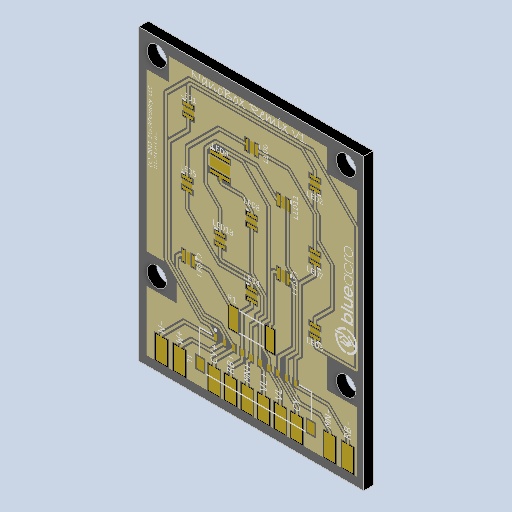
# Autodesk Inventor part: nanobox_v31_upgrade_BOARD
Saved by Autodesk Inventor 2023.2 (Build 272271030, 271C)
## iProperties
Created: 2023-03-08
Part Number: nanobox_v31_upgrade_BOARD
Material: Generic
Document SubType Name: Modeling
Designer: atrus
Density: 1 g/cm^3
Appearance: BoardColor
Author: atrus
Autodesk Inventor part; units mm, degrees
ref_plane "YZ Plane" through (0, 0, 0) normal (1, 0, 0) x (0, 1, 0)
ref_plane "XZ Plane" through (0, 0, 0) normal (0, 1, 0) x (-1, 0, 0)
ref_plane "BoardFrontPlane" through (0, 0, 0) normal (0, 0, 1) x (1, 0, 0)
sketch "Sketch1" plane through (0, 0, 0) normal (0, 0, 1) x (1, 0, 0)
  line L0 (27.9236, 28.9773) -> (27.9236, 77.9773)
  line L1 (27.9236, 77.9773) -> (65.9236, 77.9773)
  line L2 (65.9236, 77.9773) -> (65.9236, 28.9773)
  line L3 (65.9236, 28.9773) -> (27.9236, 28.9773)
  constraints: 8 end point
extrude "BoardOutline" add sketch "Sketch1" along normal blind 1.594
sketch "img_Top" plane through (0, 0, 1.594) normal (0, 0, 1) x (1, 0, 0)
  line L0 (27.9236, 77.9773) -> (65.9246, 77.9773) construction
  line L1 (65.9246, 77.9773) -> (65.9246, 28.9773) construction
  line L2 (65.9246, 28.9773) -> (27.9236, 28.9773) construction
  line L3 (27.9236, 28.9773) -> (27.9236, 77.9773) construction
  constraints: 2 other
decal "Decal_Top"
sketch "img_Bottom" plane through (0, 0, -1.594) normal (0, 0, -1) x (1, 0, 0)
  line L0 (27.9236, -28.9773) -> (65.9246, -28.9773) construction
  line L1 (65.9246, -28.9773) -> (65.9246, -77.9773) construction
  line L2 (65.9246, -77.9773) -> (27.9236, -77.9773) construction
  line L3 (27.9236, -77.9773) -> (27.9236, -28.9773) construction
  constraints: 2 other
decal "Decal_Bottom"
sketch "Sketch4" plane through (0, 0, 1.594) normal (0, 0, 1) x (1, 0, 0)
  point P0 (62.94, 42.86)
hole "Free-18" at (62.94, 42.86, 1.594) direction (0, 0, -1) diameter 3.2639 end through all
sketch "Sketch5" plane through (0, 0, 1.594) normal (0, 0, 1) x (1, 0, 0)
  point P0 (30.94, 42.86)
hole "Free-19" at (30.94, 42.86, 1.594) direction (0, 0, -1) diameter 3.2639 end through all
sketch "Sketch6" plane through (0, 0, 1.594) normal (0, 0, 1) x (1, 0, 0)
  point P0 (62.94, 75.21)
hole "Free-17" at (62.94, 75.21, 1.594) direction (0, 0, -1) diameter 3.2639 end through all
sketch "Sketch7" plane through (0, 0, 1.594) normal (0, 0, 1) x (1, 0, 0)
  point P0 (30.94, 75.21)
hole "Free-16" at (30.94, 75.21, 1.594) direction (0, 0, -1) diameter 3.2639 end through all
body "Solid1"
